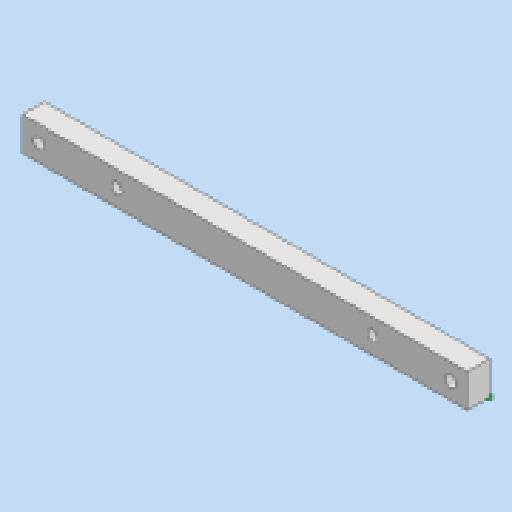
# Autodesk Inventor part: seatButtSidePlate
Saved by Autodesk Inventor 2023 (Build 270158000, 158)
## iProperties
Created: 2026-03-22
Part Number: seatButtSidePlate
Material: Generic
Document SubType Name: Modeling
Designer: Nathann
Density: 1 g/cm^3
Appearance: Default
Author: Nathann
Autodesk Inventor part; units mm, degrees
ref_plane "YZ Plane" through (0, 0, 0) normal (1, 0, 0) x (0, 1, 0)
ref_plane "XZ Plane" through (0, 0, 0) normal (0, 1, 0) x (-1, 0, 0)
ref_plane "XY Plane" through (0, 0, 0) normal (0, 0, 1) x (1, 0, 0)
sketch "Sketch1" plane through (0, 0, 0) normal (0, 0, 1) x (1, 0, 0)
  line L0 (0, 0) -> (-400, 0)
  line L1 (-400, 0) -> (-400, 30)
  line L2 (-400, 30) -> (0, 30)
  line L3 (0, 30) -> (0, 0)
  circle A0 centre (-15, 15) radius 5
  circle A1 centre (-85, 15) radius 5
  circle A2 centre (-315, 15) radius 5
  circle A3 centre (-385, 15) radius 5
  dimension "d0" = 400
  dimension "d1" = 30
  dimension "d2" = 10
  dimension "d3" = 10
  dimension "d4" = 10
  dimension "d5" = 10
  dimension "d6" = 15
  dimension "d7" = 15
  dimension "d8" = 15
  dimension "d9" = 70
  dimension "d10" = 15
  dimension "d11" = 15
  dimension "d12" = 70
  dimension "d13" = 15
  constraints: 8 end point, 4 centre point, 2 parallel, 1 horizontal, 1 perpendicular
  measures "d0" distance of L1.end L2.end
  measures "d1" distance between parallel lines of L2 L0
  measures "d2" diameter of A0
  measures "d3" diameter of A1
  measures "d4" diameter of A2
  measures "d5" diameter of A3
  measures "d6" distance from line of L3 A0.centre
  measures "d7" distance from line of L0 A0.centre
  measures "d8" distance from line of L0 A1.centre
  measures "d9" distance of A0.centre A1.centre
  measures "d10" distance from line of L1 A3.centre
  measures "d11" distance from line of L0 A3.centre
  measures "d12" distance of A3.centre A2.centre
  measures "d13" distance from line of L0 A2.centre
sketch "Sketch2" plane through (0, 0, 0) normal (0, 0, 1) x (1, 0, 0)
  point P0 (0, 0)
extrude "Extrusion1" add sketch "Sketch1" along normal blind 20
body "Solid1"
